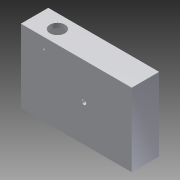
# Autodesk Inventor part: aaxaProjector01
Saved by Autodesk Inventor 2012 (Build 160160000, 160)
## iProperties
Created: 2014-06-12
Part Number: aaxaProjector01
Material: ABS Plastic
Document SubType Name: Modeling
Designer: Byron
Density: 1.06 g/cm^3
Mass: 629.203 g
Surface Area: 513.74 cm^2
Volume: 593.588 cm^3
Author: Byron
Autodesk Inventor part; units mm, degrees
ref_plane "YZ Plane" through (0, 0, 0) normal (1, 0, 0) x (0, 1, 0)
ref_plane "XZ Plane" through (0, 0, 0) normal (0, 1, 0) x (-1, 0, 0)
ref_plane "XY Plane" through (0, 0, 0) normal (0, 0, 1) x (1, 0, 0)
sketch "Sketch1" plane through (0, 0, 0) normal (0, 0, 1) x (1, 0, 0)
  line L0 (0, 0) -> (153.9875, 0)
  line L1 (153.9875, 0) -> (153.9875, 101.6)
  line L2 (153.9875, 101.6) -> (0, 101.6)
  line L3 (0, 101.6) -> (0, 0)
  dimension "d0" = 153.9875
  dimension "d1" = 101.6
  constraints: 8 end point, 2 parallel, 1 horizontal, 1 perpendicular
  measures "d0" distance of L2.end L1.end
  measures "d1" distance of L1.end L0.end
extrude "Extrusion1" add sketch "Sketch1" along normal blind 38.1
sketch "Sketch2" plane through (0, 101.6, 0) normal (0, 1, 0) x (1, 0, 0)
  line L0 (0, -38.1) -> (153.9875, -38.1) projected
  line L1 (0, 0) -> (0, -38.1) projected
  circle A0 centre (31.75, -19.05) radius 10.4767
  dimension "d4" = 31.75
  dimension "d5" = 19.05
  constraints: 1 centre point
  measures "d4" distance from line of L1 A0.centre
  measures "d5" distance from line of L0 A0.centre
extrude "Extrusion2" cut sketch "Sketch2" against normal blind 6.35
sketch "Sketch3" plane through (0, 0, 38.1) normal (0, 0, 1) x (1, 0, 0)
  line L0 (0, 0) -> (0, 101.6) projected
  line L1 (0, 101.6) -> (153.9875, 101.6) projected
  circle A0 centre (87.63, 50.8) radius 3.175
  dimension "d8" = 6.35
  dimension "d9" = 87.63
  dimension "d10" = 50.8
  constraints: 1 centre point
  measures "d8" diameter of A0
  measures "d9" distance from line of L0 A0.centre
  measures "d10" distance from line of L1 A0.centre
extrude "Extrusion3" cut sketch "Sketch3" against normal blind 9.525
sketch "Sketch4" plane through (0, 0, 38.1) normal (0, 0, 1) x (1, 0, 0)
  line L0 (42.2267, 95.25) -> (21.2733, 95.25) projected
  line L1 (31.75, 95.25) -> (31.75, 50.8) construction
  circle A0 centre (31.75, 86.77) radius 1.27
  dimension "d13" = 2.54
  constraints: 2 end point, 1 centre point, 1 midpoint, 1 perpendicular, 1 point on line
  measures "d13" diameter of A0
extrude "Extrusion4" cut sketch "Sketch4" against normal blind 25.4
body "Solid1"
